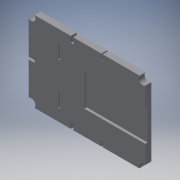
# Autodesk Inventor part: Каркас
Saved by Autodesk Inventor 2019 (Build 230136000, 136)
## iProperties
Created: 2020-05-20
Part Number: Каркас
Material: Типовые
Document SubType Name: Modeling
Designer: Surflay
Density: 1 g/cm^3
Appearance: По умолчанию
Author: Surflay
Autodesk Inventor part; units mm, degrees
ref_plane "YZ Plane" through (0, 0, 0) normal (1, 0, 0) x (0, 1, 0)
ref_plane "XZ Plane" through (0, 0, 0) normal (0, 1, 0) x (-1, 0, 0)
ref_plane "XY Plane" through (0, 0, 0) normal (0, 0, 1) x (1, 0, 0)
sketch "Эскиз1" plane through (0, 0, 0) normal (0, 0, 1) x (1, 0, 0)
  line L0 (174.3111, 41.624) -> (229.3111, 41.624) projected
  line L1 (229.3111, 41.624) -> (229.3111, 31.624) projected
  line L2 (229.3111, 31.624) -> (174.3111, 31.624) projected
  line L3 (174.3111, 41.624) -> (174.3111, 31.624) projected
  line L4 (149.3111, 46.624) -> (159.3111, 46.624) projected
  line L5 (149.3111, 46.624) -> (149.3111, 86.624) projected
  line L6 (149.3111, 86.624) -> (159.3111, 86.624) projected
  line L7 (159.3111, 86.624) -> (159.3111, 46.624) projected
  line L8 (134.3111, 31.624) -> (134.3111, 41.624) projected
  line L9 (134.3111, 31.624) -> (79.3111, 31.624) projected
  line L10 (79.3111, 31.624) -> (79.3111, 41.624) projected
  line L11 (79.3111, 41.624) -> (134.3111, 41.624) projected
  line L12 (251.3111, -20.5639) -> (251.3111, 93.8118) projected
  arc A0 (241.499, 103.624) -> (251.3111, 93.8118) centre (247.0611, 99.374) ccw projected
  line L13 (241.499, 103.624) -> (180.3111, 103.624) projected
  line L14 (180.3111, 103.624) -> (180.3111, 94.124) projected
  line L15 (180.3111, 94.124) -> (178.3111, 94.124) projected
  line L16 (178.3111, 94.124) -> (178.3111, 103.624) projected
  line L17 (178.3111, 103.624) -> (130.3111, 103.624) projected
  line L18 (130.3111, 103.624) -> (130.3111, 94.124) projected
  line L19 (130.3111, 94.124) -> (128.3111, 94.124) projected
  line L20 (128.3111, 94.124) -> (128.3111, 103.624) projected
  line L21 (128.3111, 103.624) -> (67.1233, 103.624) projected
  arc A1 (57.3111, 93.8118) -> (67.1233, 103.624) centre (61.5611, 99.374) ccw projected
  line L22 (57.3111, -20.5639) -> (57.3111, 93.8118) projected
  arc A2 (67.1233, -30.376) -> (57.3111, -20.5639) centre (61.5611, -26.126) ccw projected
  line L23 (128.3111, -30.376) -> (67.1233, -30.376) projected
  line L24 (128.3111, -30.376) -> (128.3111, -20.876) projected
  line L25 (128.3111, -20.876) -> (130.3111, -20.876) projected
  line L26 (130.3111, -20.876) -> (130.3111, -30.376) projected
  line L27 (178.3111, -30.376) -> (130.3111, -30.376) projected
  line L28 (178.3111, -30.376) -> (178.3111, -20.876) projected
  line L29 (178.3111, -20.876) -> (180.3111, -20.876) projected
  line L30 (180.3111, -20.876) -> (180.3111, -30.376) projected
  line L31 (241.499, -30.376) -> (180.3111, -30.376) projected
  arc A3 (251.3111, -20.5639) -> (241.499, -30.376) centre (247.0611, -26.126) ccw projected
  circle A4 centre (229.3111, 86.624) radius 5 projected
  circle A5 centre (79.3111, -13.376) radius 5 projected
  circle A6 centre (79.3111, 86.624) radius 5 projected
  circle A7 centre (229.3111, -13.376) radius 5 projected
  line L32 (159.3111, 26.624) -> (149.3111, 26.624) projected
  line L33 (159.3111, 26.624) -> (159.3111, -13.376) projected
  line L34 (159.3111, -13.376) -> (149.3111, -13.376) projected
  line L35 (149.3111, -13.376) -> (149.3111, 26.624) projected
  line L36 (241.499, 103.624) -> (67.1233, 103.624)
  line L37 (57.3111, 93.8118) -> (57.3111, -20.5639)
  line L38 (67.1233, -30.376) -> (241.499, -30.376)
  line L39 (251.3111, -20.5639) -> (251.3111, 93.8118)
  arc A8 (251.3111, -20.5639) -> (241.499, -30.376) centre (247.0611, -26.126) ccw
  arc A9 (67.1233, -30.376) -> (57.3111, -20.5639) centre (61.5611, -26.126) ccw
  arc A10 (57.3111, 93.8118) -> (67.1233, 103.624) centre (61.5611, 99.374) ccw
  arc A11 (241.499, 103.624) -> (251.3111, 93.8118) centre (247.0611, 99.374) ccw
  line L40 (57.3111, 35.624) -> (57.3111, 37.624) construction
  line L41 (251.3111, 35.624) -> (251.3111, 37.624) construction
  line L42 (181.3111, -30.376) -> (177.3111, -30.376)
  line L43 (177.3111, -30.376) -> (177.3111, -20.376)
  line L44 (177.3111, -20.376) -> (181.3111, -20.376)
  line L45 (181.3111, -20.376) -> (181.3111, -30.376)
  line L46 (131.3111, -30.376) -> (127.3111, -30.376)
  line L47 (127.3111, -30.376) -> (127.3111, -20.376)
  line L48 (127.3111, -20.376) -> (131.3111, -20.376)
  line L49 (131.3111, -20.376) -> (131.3111, -30.376)
  line L50 (57.3111, 34.624) -> (67.3111, 34.624)
  line L51 (67.3111, 34.624) -> (67.3111, 38.624)
  line L52 (67.3111, 38.624) -> (57.3111, 38.624)
  line L53 (57.3111, 38.624) -> (57.3111, 34.624)
  line L54 (131.3111, 103.624) -> (127.3111, 103.624)
  line L55 (127.3111, 103.624) -> (127.3111, 93.624)
  line L56 (127.3111, 93.624) -> (131.3111, 93.624)
  line L57 (131.3111, 93.624) -> (131.3111, 103.624)
  line L58 (181.3111, 103.624) -> (177.3111, 103.624)
  line L59 (177.3111, 103.624) -> (177.3111, 93.624)
  line L60 (177.3111, 93.624) -> (181.3111, 93.624)
  line L61 (181.3111, 93.624) -> (181.3111, 103.624)
  line L62 (251.3111, 38.624) -> (241.3111, 38.624)
  line L63 (241.3111, 38.624) -> (241.3111, 34.624)
  line L64 (241.3111, 34.624) -> (251.3111, 34.624)
  line L65 (251.3111, 34.624) -> (251.3111, 38.624)
  point P0 (0, 0)
  point P1 (154.3111, 103.624)
  point P2 (154.3111, -30.376)
  point P3 (57.3111, 36.624)
  point P4 (251.3111, 36.624)
  point P5 (179.3111, -20.376)
  point P6 (179.3111, -20.876)
  point P7 (129.3111, -20.376)
  point P8 (129.3111, -20.876)
  point P9 (67.3111, 36.624)
  point P10 (66.8111, 36.624)
  point P11 (129.3111, 93.624)
  point P12 (129.3111, 94.124)
  point P13 (179.3111, 93.624)
  point P14 (179.3111, 94.124)
  point P15 (241.3111, 36.624)
  point P16 (241.8111, 36.624)
  dimension "d0" = 4
  dimension "d1" = 10
  dimension "d2" = 10
  dimension "d3" = 4
  dimension "d4" = 10
  dimension "d5" = 4
  dimension "d6" = 10
  dimension "d7" = 4
  dimension "d8" = 4
  dimension "d9" = 10
  dimension "d10" = 10
  dimension "d11" = 4
  constraints: 60 end point, 18 midpoint, 16 point on circle, 14 parallel, 7 horizontal, 7 perpendicular, 6 point on line, 4 centre point, 4 vertical alignment, 2 concentric, 2 horizontal alignment, 2 vertical, 1 coincident
  measures "d0" distance of L43.end L44.end
  measures "d1" distance of L42.end L43.end
  measures "d2" distance of L46.end L47.end
  measures "d3" distance of L47.end L48.end
  measures "d4" distance of L50.start L50.end
  measures "d5" distance of L50.end L51.end
  measures "d6" distance of L54.end L55.end
  measures "d7" distance of L55.end L56.end
  measures "d8" distance of L59.end L60.end
  measures "d9" distance of L58.end L59.end
  measures "d10" distance of L62.start L62.end
  measures "d11" distance of L62.end L63.end
extrude "Выдавливание1" add sketch "Эскиз1" along normal blind 10 contours L0 L1 L2 L3 | L5 L6 L7 L4 | L9 L10 L11 L8 | A3 L31 L45 L44 L43 L27 L49 L48 L47 L23 A2 L22 L50 L51 L52 A1 L21 L55 L56 L57 L17 L59 L60 L61 L13 A0 L12 L62 L63 L64 | L64 L63 L62 L12 | L31 L30 L29 L28 L27 L43 L44 L45 | L61 L60 L59 L17 L16 L15 L14 L13 | A4 | A5 | A6 | A7 | L33 L34 L35 L32
sketch "Эскиз2" plane through (0, 0, 10) normal (0, 0, 1) x (1, 0, 0)
  line L0 (251.3111, 9.954) -> (149.7111, 9.954)
  line L1 (149.7111, 9.954) -> (149.7111, 63.294)
  line L2 (149.7111, 63.294) -> (251.3111, 63.294)
  line L3 (251.3111, 63.294) -> (251.3111, 9.954)
  line L4 (251.3111, -20.5639) -> (251.3111, 35.624) projected
  line L5 (251.3111, 37.624) -> (251.3111, 93.8118) projected
  line L6 (251.3111, 35.624) -> (251.3111, 37.624) construction
  line L7 (154.7911, 9.954) -> (251.3111, 9.954) projected
  point P0 (0, 0)
  point P1 (251.3111, 36.624)
  dimension "d14" = 101.6
  dimension "d15" = 53.34
  constraints: 10 end point, 2 midpoint, 2 parallel, 1 horizontal, 1 perpendicular, 1 vertical
  measures "d14" distance of L0.start L0.end
  measures "d15" distance of L0.end L1.end
extrude "Выдавливание2" cut sketch "Эскиз2" against normal blind 4
sketch "Эскиз9" plane through (0, 0, 10) normal (0, 0, 1) x (1, 0, 0)
  line L0 (109.3111, 83.624) -> (107.3111, 83.624) projected
  line L1 (109.3111, 62.124) -> (109.3111, 81.124) projected
  line L2 (107.3111, 62.124) -> (107.3111, 81.124) projected
  line L3 (109.3111, 59.624) -> (107.3111, 59.624) projected
  line L4 (106.4111, 62.5941) -> (106.4111, 64.4694) projected
  line L5 (106.4111, 69.3382) -> (106.4111, 70.0888) projected
  line L6 (106.4111, 77.7718) -> (106.4111, 78.6108) projected
  line L7 (106.4111, 79.5822) -> (106.4111, 80.2887) projected
  line L8 (109.3111, 83.624) -> (106.4111, 83.624)
  line L9 (106.4111, 83.624) -> (106.4111, 59.624)
  line L10 (106.4111, 59.624) -> (109.3111, 59.624)
  line L11 (109.3111, 59.624) -> (109.3111, 83.624)
  point P0 (0, 0)
  constraints: 8 end point, 2 parallel, 1 horizontal, 1 perpendicular
extrude "Выдавливание11" cut sketch "Эскиз9" against normal blind 4
pattern_linear "Прямоуг.массив1" count 2 spacing 70 along (0, -1, 0) of "Выдавливание11"
equation "\"d2\" = d1"
equation "\"d3\" = d0"
equation "\"d4\" = d2"
equation "\"d5\" = d3"
equation "\"d6\" = d4"
equation "\"d7\" = d5"
equation "\"d8\" = d7"
equation "\"d9\" = d6"
equation "\"d10\" = d1"
equation "\"d11\" = d0"
